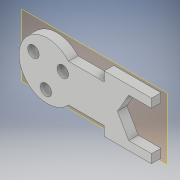
# Autodesk Inventor part: Деталь_1
Saved by Autodesk Inventor 2019.3 (Build 233278000, 278)
## iProperties
Created: 2020-03-02
Part Number: Деталь_1
Material: Типовые
Document SubType Name: Modeling
Designer: Diana
Density: 1 g/cm^3
Appearance: По умолчанию
Author: Diana
Autodesk Inventor part; units mm, degrees
ref_plane "YZ Plane" through (0, 0, 0) normal (1, 0, 0) x (0, 1, 0)
ref_plane "XZ Plane" through (0, 0, 0) normal (0, 1, 0) x (-1, 0, 0)
sketch "Эскиз1" plane through (0, 0, 0) normal (0, 0, 1) x (1, 0, 0)
  arc A0 (11.1803, 10) -> (11.1803, -10) centre (0, 0) ccw
  line L0 (30, 15) -> (55, 15)
  line L1 (55, 15) -> (55, -15)
  line L2 (55, -15) -> (30, -15)
  line L3 (30, -15) -> (30, 15)
  line L4 (11.1803, 10) -> (30, 10)
  line L5 (11.1803, -10) -> (30, -10)
  line L6 (37, 0) -> (43, 10.3923)
  line L7 (43, 10.3923) -> (55, 10.3923)
  line L8 (55, 10.3923) -> (61, 0)
  line L9 (61, 0) -> (55, -10.3923)
  line L10 (55, -10.3923) -> (43, -10.3923)
  line L11 (43, -10.3923) -> (37, 0)
  line L12 (-7.3724, 5.1622) -> (0, 0)
  line L13 (0, 8.3003) -> (0, 0)
  circle A1 centre (-7.3724, 5.1622) radius 3
  circle A2 centre (8.1568, 3.8036) radius 3
  circle A3 centre (-0.7844, -8.9658) radius 3
  point P0 (49, 0)
  dimension "d0" = 15
  dimension "d1" = 25
  dimension "d2" = 30
  dimension "d5" = 15
  dimension "d6" = 30
  dimension "d7" = 10
  dimension "d8" = 24
  dimension "d9" = 9
  dimension "d11" = 55
  dimension "d12" = 6
  dimension "d15" = 360
  constraints: 28 end point, 9 coincident, 4 centre point, 4 parallel, 4 point on line, 2 horizontal, 2 point on circle, 1 horizontal alignment, 1 perpendicular, 1 vertical, 28 other
  measures "d0" radius of A0
  measures "d1" distance of L1.end L2.end
  measures "d2" distance of L0.end L1.end
  measures "d5" distance from line of L0 point (0, 0)
  measures "d6" horizontal distance of L2.end point (0, 0)
  measures "d7" distance from line of L4 point (0, 0)
  measures "d8" distance of L8.end L6.start
  measures "d9" distance of point (0, 0) L12.start
  measures "d11" angle of L13 L12
  measures "d12" diameter of A1
extrude "Выдавливание1" add sketch "Эскиз1" along normal blind 5 contours L4 L3 L5 A0 | L3 L0 L1 L7 L6 L11 L10 L2
